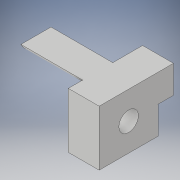
# Autodesk Inventor part: end peice for slides
Saved by Autodesk Inventor 2019 (Build 230136000, 136)
## iProperties
Created: 2019-05-04
Part Number: end peice for slides
Material: Generic
Document SubType Name: Modeling
Designer: User
Density: 1 g/cm^3
Appearance: Default
Author: User
Autodesk Inventor part; units mm, degrees
ref_plane "YZ Plane" through (0, 0, 0) normal (1, 0, 0) x (0, 1, 0)
ref_plane "XZ Plane" through (0, 0, 0) normal (0, 1, 0) x (-1, 0, 0)
ref_plane "XY Plane" through (0, 0, 0) normal (0, 0, 1) x (1, 0, 0)
sketch "Sketch1" plane through (0, 0, 0) normal (1, 0, 0) x (0, 1, 0)
  line L0 (0, 0) -> (11.4, 0)
  line L1 (11.4, 0) -> (11.4, -12.1)
  line L2 (11.4, -12.1) -> (0, -12.1)
  line L3 (0, -12.1) -> (0, 0)
  arc A0 (11.4, -2.9512) -> (11.4, -9.1488) centre (12.8006, -6.05) ccw
  point P0 (3.5, -5)
  dimension "d0" = 11.4
  dimension "d1" = 12.1
  dimension "d2" = 6.1976
  dimension "d3" = 2.9512
  dimension "d29" = 2
  constraints: 8 end point, 2 parallel, 2 point on circle, 2 point on line, 1 centre point, 1 horizontal, 1 perpendicular
  measures "d0" distance of L1.end L2.end
  measures "d1" distance of L0.end L1.end
  measures "d2" distance of A0.end A0.start
  measures "d3" distance of L1.end A0.end
  measures "d29" distance edge to line of A0 L1
extrude "Extrusion1" add sketch "Sketch1" along normal blind 6.35
extrude "Extrusion2" add sketch "Sketch1" against normal blind 12.7 contours L1 A0
sketch "Sketch3" plane through (0, 0, 0) normal (-1, 0, 0) x (0, 0, 1)
  line L0 (0, 11.4) -> (0, 0) projected
  line L1 (0, 0) -> (-12.1, 0) projected
  point P0 (-6.05, 5.7)
  dimension "d19" = 12.1
  dimension "d20" = 6.05
  dimension "d30" = 11.4
  dimension "d31" = 5.7
  measures "d19" distance of L0.end L1.end
  measures "d20" distance from line of L0 point (-6.05, 5.7)
  measures "d30" distance of L0.start L0.end
  measures "d31" distance from line of L1 point (-6.05, 5.7)
hole "Hole2" at (0, 5.7, -6.05) direction (1, 0, 0) diameter 4 end through all
sketch "Sketch9" plane through (0, 0, -12.1) normal (0, 0, -1) x (-1, 0, 0)
  line L0 (-6.35, 0) -> (-6.35, 11.4) projected
  line L1 (0, 0) -> (0, 11.4) projected
  line L2 (-6.35, 11.4) -> (0, 11.4)
  line L3 (0, 11.4) -> (0, 5.7)
  line L4 (0, 5.7) -> (-6.35, 5.7)
  line L5 (-6.35, 5.7) -> (-6.35, 11.4)
  dimension "d70" = 11.4
  dimension "d71" = 5.7
  constraints: 8 end point, 2 parallel, 1 horizontal, 1 midpoint, 1 perpendicular
  measures "d70" distance of L0.start L0.end
  measures "d71" distance between parallel lines of L2 L4
extrude "Extrusion10" add sketch "Sketch9" along normal blind 3.175
sketch "Sketch10" plane through (0, 0, -15.275) normal (0, 0, -1) x (-1, 0, 0)
  circle A0 centre (-3.175, 8.55) radius 1.9939
  line L0 (-6.35, 11.4) -> (-6.35, 5.7) projected
  line L1 (0, 11.4) -> (-6.35, 11.4) projected
  point P0 (0, 0)
  dimension "d74" = 6.35
  dimension "d75" = 5.7
  dimension "d76" = 2.85
  dimension "d77" = 3.175
  dimension "d80" = 3.9878
  constraints: 1 centre point
  measures "d74" distance of L1.start L0.start
  measures "d75" distance of L0.start L0.end
  measures "d76" distance from line of L1 A0.centre
  measures "d77" distance from line of L0 A0.centre
  measures "d80" diameter of A0
extrude "Extrusion11" cut sketch "Sketch10" against normal up to surface (3.175 mm away)
thread "Thread3" size "M4x0.7" class "6H" standard "ISO Metric profile" full length
equation "\"d3\" = -0.5 * d2 + 0.5 * d1"
equation "\"d20\" = 0.5 * d19"
equation "\"d31\" = 0.5 * d30"
equation "\"d71\" = 0.5 * d70"
equation "\"d76\" = 0.5 * d75"
equation "\"d77\" = 0.5 * d74"
body "Solid1"
